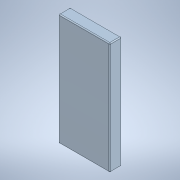
# Autodesk Inventor part: magnet_11x24-x2_5
Saved by Autodesk Inventor 2022 (Build 260153000, 153)
## iProperties
Created: 2025-01-12
Part Number: magnet_11x24-x2_5
Material: Generic
Document SubType Name: Modeling
Designer: Home
Density: 1 g/cm^3
Appearance: Steel Blue
Author: Home
Autodesk Inventor part; units mm, degrees
ref_plane "YZ Plane" through (0, 0, 0) normal (1, 0, 0) x (0, 1, 0)
ref_plane "XZ Plane" through (0, 0, 0) normal (0, 1, 0) x (-1, 0, 0)
ref_plane "XY Plane" through (0, 0, 0) normal (0, 0, 1) x (1, 0, 0)
sketch "Sketch1" plane through (0, 0, 0) normal (0, 0, 1) x (1, 0, 0)
  line L0 (-5.5, -12) -> (5.5, -12)
  line L1 (5.5, -12) -> (5.5, 12)
  line L2 (5.5, 12) -> (-5.5, 12)
  line L3 (-5.5, 12) -> (-5.5, -12)
  line L4 (-5.5, -12) -> (5.5, 12) construction
  line L5 (5.5, -12) -> (-5.5, 12) construction
  point P0 (0, 0)
  dimension "d0" = 11
  dimension "d1" = 24
  constraints: 12 end point, 2 midpoint, 2 parallel, 1 horizontal, 1 perpendicular
  measures "d0" distance of L2.end L1.end
  measures "d1" distance of L1.end L0.end
extrude "Extrusion1" add sketch "Sketch1" along normal blind 2.5
fillet "Fillet1" radius 0.2 12 edges at (-5.5, 12, 1.25) (0, 12, 0) (0, 12, 2.5) (5.5, 12, 1.25) (5.5, -12, 1.25) (0, -12, 2.5) (0, -12, 0) (-5.5, -12, 1.25) (-5.5, 0, 2.5) (5.5, 0, 2.5) (5.5, 0, 0) (-5.5, 0, 0)
body "Solid1"
